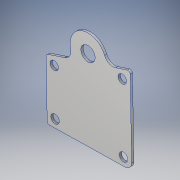
# Autodesk Inventor part: Column Plate
Saved by Autodesk Inventor 2019.4 (Build 234330000, 330)
## iProperties
Created: 2020-01-18
Part Number: Column Plate
Material: Aluminum 6061
Document SubType Name: Modeling
Designer: admin
Density: 2.7 g/cm^3
Appearance: Aluminum - Flat
Mass: 599.617 g
Surface Area: 961.226 cm^2
Volume: 222.08 cm^3
Author: admin
Autodesk Inventor part; units mm, degrees
ref_plane "YZ Plane" through (0, 0, 0) normal (1, 0, 0) x (0, 1, 0)
ref_plane "XZ Plane" through (0, 0, 0) normal (0, 1, 0) x (-1, 0, 0)
ref_plane "XY Plane" through (0, 0, 0) normal (0, 0, 1) x (1, 0, 0)
sketch "Sketch1" plane through (0, 0, 0) normal (0, 0, 1) x (1, 0, 0)
  line L0 (-192.5097, 176.4187) -> (-194.9395, 310.4801)
  line L1 (-194.9395, 310.4801) -> (-6.7464, 372.2232)
  circle A0 centre (-176.7016, 297.5197) radius 9.5
  circle A1 centre (-24.3016, 347.5197) radius 9.5
  circle A2 centre (-174.8388, 194.7419) radius 9.5
  circle A3 centre (-79, 86.5538) radius 88.9 construction
  line L2 (-192.5097, 176.4187) -> (-3.2597, 179.8488)
  line L3 (-3.2597, 179.8488) -> (-6.7464, 372.2232)
  circle A4 centre (-21.5829, 197.5197) radius 9.5
  circle A5 centre (-95, 255.4656) radius 88.9 construction
  circle A6 centre (-101.1464, 358.0912) radius 16
  circle A7 centre (-101.1464, 358.0912) radius 40
  line L4 (-101.1464, 358.0912) -> (-97.8847, 178.1338) construction
  point P0 (0, 0)
  dimension "d22" = 19
  dimension "d23" = 19
  dimension "d24" = 18
  dimension "d25" = 18
  dimension "d27" = 18
  dimension "d28" = 19
  dimension "d29" = 18
  dimension "d35" = 177.8
  dimension "d38" = 19
  dimension "d40" = 18
  dimension "d41" = 152.4
  dimension "d42" = 18
  dimension "d43" = 50
  dimension "d45" = 177.8
  dimension "d46" = 100
  dimension "d51" = 32
  dimension "d52" = 80
  dimension "d56" = 18
  dimension "d57" = 18
  constraints: 10 end point, 8 centre point, 3 perpendicular, 1 coincident, 1 midpoint, 1 point on line, 1 tangent
  measures "d22" diameter of A0
  measures "d23" diameter of A1
  measures "d24" distance from line of L0 A0.centre
  measures "d25" distance from line of L1 A0.centre
  measures "d27" distance from line of L1 A1.centre
  measures "d28" diameter of A2
  measures "d29" distance from line of L0 A2.centre
  measures "d35" diameter of A3
  measures "d38" diameter of A4
  measures "d40" distance from line of L3 A4.centre
  measures "d41" horizontal distance of A1.centre A0.centre
  measures "d42" distance from line of L3 A1.centre
  measures "d43" vertical distance of A1.centre A0.centre
  measures "d45" diameter of A5
  measures "d46" vertical distance of A4.centre A0.centre
  measures "d51" diameter of A6
  measures "d52" diameter of A7
  measures "d56" distance from line of L2 A2.centre
  measures "d57" distance from line of L2 A4.centre
extrude "Extrusion1" add sketch "Sketch1" along normal blind 5
fillet "Fillet1" radius 5 1 edges at (-192.5097, 176.4187, 2.5)
fillet "Fillet2" radius 15 1 edges at (-3.2597, 179.8488, 2.5)
fillet "Fillet4" radius 5 2 edges at (-194.9395, 310.4801, 2.5) (-6.7464, 372.2232, 2.5)
fillet "Fillet5" radius 20 2 edges at (-130.9924, 331.4601, 2.5) (-61.3248, 354.3169, 2.5)
body "Solid1"
